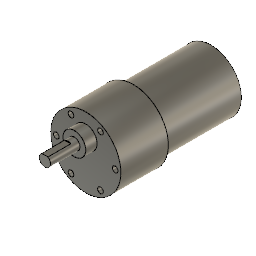
MOTOR_SPG30E-60K v1 (Autodesk Fusion 360 design; units mm, degrees)
Autodesk Fusion 360 part; units mm, degrees
sketch "Sketch1" plane through (0, 0, 0) normal (0, 1, 0) x (1, 0, 0)
  circle A0 centre (0, 0) radius 18.5
  circle A1 centre (0, 0) radius 16
  circle A2 centre (0, 0) radius 15.5 construction
  line L0 (-18.5, 0) -> (18.5, 0) construction
  circle A3 centre (15.5, 0) radius 1.5
  circle A4 centre (-15.5, 0) radius 1.5
  line L1 (9.25, -16.0215) -> (-9.25, 16.0215) construction
  line L2 (9.25, 16.0215) -> (-9.25, -16.0215) construction
  circle A5 centre (7.75, -13.4234) radius 1.5
  circle A6 centre (-7.75, -13.4234) radius 1.5
  circle A7 centre (-7.75, 13.4234) radius 1.5
  circle A8 centre (7.75, 13.4234) radius 1.5
  line L3 (-14.3875, -7) -> (14.3875, -7) construction
  circle A9 centre (0, -7) radius 3
  circle A10 centre (0, -7) radius 6
  line L4 (-1.6583, -9.5) -> (1.6583, -9.5)
  dimension "d2" = 37
  dimension "d3" = 32
  dimension "d5" = 31
  dimension "d6" = 3
  dimension "d7" = 3
  dimension "d8" = 60
  dimension "d9" = 120
  dimension "d10" = 3
  dimension "d11" = 3
  dimension "d12" = 3
  dimension "d13" = 3
  dimension "d14" = 7
  dimension "d15" = 6
  dimension "d16" = 12
  dimension "d31" = 5.5
  constraint concentric A0 A1
  constraint coincident A0 L0.start
  constraint horizontal L0
  constraint midpoint A0.centre L0
  constraint coincident A0.centre A1.centre
  constraint coincident A2 A3.centre
  constraint coincident L0 A3.centre
  constraint coincident A2 A4.centre
  constraint coincident L0 A4.centre
  constraint coincident A0 L1.start
  constraint coincident A0 L1.end
  constraint midpoint A0.centre L1
  constraint coincident A0 L2.start
  constraint coincident A0 L2.end
  constraint midpoint A0.centre L2
  constraint coincident A2 A5.centre
  constraint coincident L1 A5.centre
  constraint coincident A2 A6.centre
  constraint coincident L2 A6.centre
  constraint coincident A2 A7.centre
  constraint coincident L1 A7.centre
  constraint coincident A2 A8.centre
  constraint coincident A1 L3.end
  constraint horizontal L3
  constraint coincident A1 L3.start
  constraint midpoint L3 A9.centre
  constraint concentric A9 A10
  constraint coincident A9 L4.start
  constraint coincident A9 L4.end
  constraint parallel L3 L4
  measures "d2" diameter of A0
  measures "d3" diameter of A1
  measures "d5" diameter of A2
  measures "d6" diameter of A3
  measures "d7" diameter of A4
  measures "d8" angle of L0 L1
  measures "d9" angle of L1 L2
  measures "d10" diameter of A5
  measures "d11" diameter of A6
  measures "d12" diameter of A7
  measures "d13" diameter of A8
  measures "d14" distance of L0 L3
  measures "d15" diameter of A9
  measures "d16" diameter of A10
extrude "Extrude1" add sketch "Sketch1" along normal blind 25 contours A0 | A1 A3 | A1 A3 | A1 A3 A4 A5 A6 A7 A8 | A1 A8 | A1 A8 | A1 A5 | A1 A5 | A1 A7 | A1 A7 | A1 A6 | A1 A6 | A1 A4 | A1 A4 | A9 L4 | A9 L4 | A10
extrude "Extrude2" add sketch "Sketch1" along normal blind 26 from surface at 25 contours A1 A3 | A1 A3 A4 A5 A6 A7 A8 | A1 A8 | A1 A5 | A1 A7 | A1 A6 | A1 A4 | A9 L4 | A9 L4 | A10 picked at (15.3976, -0.4091) picked at (7.6973, 13.2575) picked at (7.6973, -13.2575) picked at (-7.6523, 13.282) picked at (-7.6523, -13.282) picked at (-15.3286, 0)
extrude "Extrude3" add 1 faces at (-4.5682, 51, 0.742) along direction (0, 1, 0) blind 15
extrude "Extrude4" add sketch "Sketch1" against normal blind 6 contours A9 L4 | A9 L4 | A10
extrude "Extrude5" add sketch "Sketch1" against normal blind 15.5 from surface at -6 contours A9 L4 | A9 L4
extrude "Extrude6" cut sketch "Sketch1" along normal blind 3.5 contours A1 A3 | A1 A3 | A1 A8 | A1 A8 | A1 A5 | A1 A5 | A1 A7 | A1 A7 | A1 A6 | A1 A6 | A1 A4 | A1 A4
extrude "Extrude7" cut sketch "Sketch1" along normal blind 12 from surface at -21.5 contours A9 L4 picked at (0.4253, -9.5717)
